Autodesk Inventor part; units mm, degrees
(part 2 of 2)
  spline S272 degree 2 poles (-165.9492, 93.5907) (-165.8958, 93.5647) (-165.7531, 93.5242) (-165.6883, 93.5242) knots 0 0 0 1 2 2 2
  spline S273 degree 2 poles (-165.6883, 93.5242) (-165.4922, 93.5242) (-165.2539, 93.8208) (-165.2539, 94.0915) knots 0 0 0 1 2 2 2
  spline S274 degree 2 poles (-165.2539, 94.0915) (-165.2539, 94.3557) (-165.4841, 94.6523) (-165.6883, 94.6523) knots 0 0 0 1 2 2 2
  spline S275 degree 2 poles (-165.6883, 94.6523) (-165.8115, 94.6523) (-166.0351, 94.5502) (-166.121, 94.4707) knots 0 0 0 1 2 2 2
  line L249 (-166.121, 94.4707) -> (-166.1356, 94.4707)
  line L250 (-166.1356, 94.4707) -> (-166.1356, 94.7544)
  spline S276 degree 2 poles (-166.1356, 94.7544) (-166.0984, 94.7722) (-165.9849, 94.8224) (-165.9395, 94.8338) knots 0 0 0 1 2 2 2
  spline S277 degree 2 poles (-165.9395, 94.8338) (-165.8747, 94.8532) (-165.7726, 94.8727) (-165.6932, 94.8727) knots 0 0 0 1 2 2 2
  spline S278 degree 2 poles (-167.2021, 94.6798) (-167.1713, 94.7025) (-167.0676, 94.7835) (-167.0189, 94.8079) knots 0 0 0 1 2 2 2
  spline S279 degree 2 poles (-167.0189, 94.8079) (-166.9525, 94.8435) (-166.8277, 94.8808) (-166.7142, 94.8808) knots 0 0 0 1 2 2 2
  spline S280 degree 2 poles (-166.7142, 94.8808) (-166.6219, 94.8808) (-166.4549, 94.8111) (-166.3917, 94.7479) knots 0 0 0 1 2 2 2
  spline S281 degree 2 poles (-166.3917, 94.7479) (-166.3317, 94.6863) (-166.2588, 94.5048) (-166.2588, 94.4043) knots 0 0 0 1 2 2 2
  spline S282 degree 2 poles (-166.2588, 94.4043) (-166.2588, 94.2487) (-166.3901, 94.0283) (-166.5327, 93.9651) knots 0 0 0 1 2 2 2
  spline S283 degree 2 poles (-166.5327, 93.9651) (-166.6591, 93.9067) (-167.0027, 93.863) (-167.2021, 93.8516) knots 0 0 0 1 2 2 2
  line L251 (-167.2021, 93.8516) -> (-167.2021, 93.803)
  spline S284 degree 2 poles (-167.2021, 93.803) (-167.2021, 93.7155) (-167.1486, 93.6069) (-167.1, 93.5761) knots 0 0 0 1 2 2 2
  spline S285 degree 2 poles (-167.1, 93.5761) (-167.0514, 93.5453) (-166.912, 93.5259) (-166.8374, 93.5259) knots 0 0 0 1 2 2 2
  spline S286 degree 2 poles (-166.8374, 93.5259) (-166.7499, 93.5259) (-166.5133, 93.5777) (-166.395, 93.628) knots 0 0 0 1 2 2 2
  line L252 (-166.395, 93.628) -> (-166.3804, 93.628)
  line L253 (-166.3804, 93.628) -> (-166.3804, 93.3703)
  spline S287 degree 2 poles (-166.3804, 93.3703) (-166.4501, 93.3508) (-166.711, 93.3022) (-166.839, 93.3022) knots 0 0 0 1 2 2 2
  spline S288 degree 2 poles (-166.839, 93.3022) (-166.9946, 93.3022) (-167.2069, 93.3508) (-167.2912, 93.414) knots 0 0 0 1 2 2 2
  spline S289 degree 2 poles (-167.2912, 93.414) (-167.3739, 93.4756) (-167.4549, 93.6717) (-167.4549, 93.8127) knots 0 0 0 1 2 2 2
  line L254 (-167.4549, 93.8127) -> (-167.4549, 94.8387)
  line L255 (-167.4549, 94.8387) -> (-167.2021, 94.8387)
  line L256 (-167.2021, 94.8387) -> (-167.2021, 94.6798)
  line L257 (-167.2021, 94.4691) -> (-167.2021, 94.0526)
  spline S290 degree 2 poles (-167.2021, 94.0526) (-167.1113, 94.0607) (-166.8374, 94.0882) (-166.7515, 94.1142) knots 0 0 0 1 2 2 2
  spline S291 degree 2 poles (-166.7515, 94.1142) (-166.651, 94.145) (-166.5197, 94.273) (-166.5197, 94.3865) knots 0 0 0 1 2 2 2
  spline S292 degree 2 poles (-166.5197, 94.3865) (-166.5197, 94.5161) (-166.6656, 94.6474) (-166.805, 94.6474) knots 0 0 0 1 2 2 2
  spline S293 degree 2 poles (-166.805, 94.6474) (-166.9233, 94.6474) (-167.1178, 94.5453) (-167.2021, 94.4691) knots 0 0 0 1 2 2 2
  line L258 (-169.5116, 94.8387) -> (-169.5116, 93.9699)
  spline S294 degree 2 poles (-169.5116, 93.9699) (-169.5116, 93.8662) (-169.4954, 93.6895) (-169.4695, 93.6409) knots 0 0 0 1 2 2 2
  spline S295 degree 2 poles (-169.4695, 93.6409) (-169.4436, 93.5874) (-169.3447, 93.5356) (-169.2588, 93.5356) knots 0 0 0 1 2 2 2
  spline S296 degree 2 poles (-169.2588, 93.5356) (-169.181, 93.5356) (-169.0027, 93.6312) (-168.9087, 93.722) knots 0 0 0 1 2 2 2
  spline S297 degree 2 poles (-168.9087, 93.722) (-168.9103, 93.7447) (-168.9136, 93.8079) (-168.9136, 93.85) knots 0 0 0 1 2 2 2
  line L259 (-168.9136, 93.85) -> (-168.9136, 94.8387)
  line L260 (-168.9136, 94.8387) -> (-168.6608, 94.8387)
  line L261 (-168.6608, 94.8387) -> (-168.6608, 93.9699)
  spline S298 degree 2 poles (-168.6608, 93.9699) (-168.6608, 93.8662) (-168.6445, 93.6895) (-168.6186, 93.6409) knots 0 0 0 1 2 2 2
  spline S299 degree 2 poles (-168.6186, 93.6409) (-168.5927, 93.5874) (-168.4938, 93.5356) (-168.4079, 93.5356) knots 0 0 0 1 2 2 2
  spline S300 degree 2 poles (-168.4079, 93.5356) (-168.3269, 93.5356) (-168.147, 93.6377) (-168.0627, 93.7171) knots 0 0 0 1 2 2 2
  line L262 (-168.0627, 93.7171) -> (-168.0627, 94.8387)
  line L263 (-168.0627, 94.8387) -> (-167.8099, 94.8387)
  line L264 (-167.8099, 94.8387) -> (-167.8099, 93.3378)
  line L265 (-167.8099, 93.3378) -> (-168.0627, 93.3378)
  line L266 (-168.0627, 93.3378) -> (-168.0627, 93.5032)
  spline S301 degree 2 poles (-168.0627, 93.5032) (-168.1616, 93.4043) (-168.3561, 93.2957) (-168.4727, 93.2957) knots 0 0 0 1 2 2 2
  spline S302 degree 2 poles (-168.4727, 93.2957) (-168.6056, 93.2957) (-168.8115, 93.4173) (-168.865, 93.555) knots 0 0 0 1 2 2 2
  spline S303 degree 2 poles (-168.865, 93.555) (-168.98, 93.427) (-169.1972, 93.2957) (-169.3236, 93.2957) knots 0 0 0 1 2 2 2
  spline S304 degree 2 poles (-169.3236, 93.2957) (-169.4209, 93.2957) (-169.5797, 93.3557) (-169.6381, 93.4237) knots 0 0 0 1 2 2 2
  spline S305 degree 2 poles (-169.6381, 93.4237) (-169.698, 93.4918) (-169.7645, 93.696) (-169.7645, 93.85) knots 0 0 0 1 2 2 2
  line L267 (-169.7645, 93.85) -> (-169.7645, 94.8387)
  line L268 (-169.7645, 94.8387) -> (-169.5116, 94.8387)
  spline S306 degree 2 poles (-170.771, 94.8727) (-170.4112, 94.8727) (-170.0157, 94.4691) (-170.0157, 94.0964) knots 0 0 0 1 2 2 2
  spline S307 degree 2 poles (-170.0157, 94.0964) (-170.0157, 93.7301) (-170.3998, 93.2957) (-170.7094, 93.2957) knots 0 0 0 1 2 2 2
  spline S308 degree 2 poles (-170.7094, 93.2957) (-170.8488, 93.2957) (-171.0643, 93.3767) (-171.1437, 93.4626) knots 0 0 0 1 2 2 2
  spline S309 degree 2 poles (-171.1437, 93.4626) (-171.2248, 93.5485) (-171.3107, 93.7965) (-171.3107, 93.9764) knots 0 0 0 1 2 2 2
  line L269 (-171.3107, 93.9764) -> (-171.3107, 94.1142)
  line L270 (-171.3107, 94.1142) -> (-170.2718, 94.1142)
  spline S310 degree 2 poles (-170.2718, 94.1142) (-170.2718, 94.3751) (-170.5343, 94.6523) (-170.7677, 94.6523) knots 0 0 0 1 2 2 2
  spline S311 degree 2 poles (-170.7677, 94.6523) (-170.8504, 94.6523) (-171.0108, 94.615) (-171.0757, 94.5858) knots 0 0 0 1 2 2 2
  spline S312 degree 2 poles (-171.0757, 94.5858) (-171.1437, 94.5534) (-171.2377, 94.4967) (-171.2685, 94.4707) knots 0 0 0 1 2 2 2
  line L271 (-171.2685, 94.4707) -> (-171.2831, 94.4707)
  line L272 (-171.2831, 94.4707) -> (-171.2831, 94.7463)
  spline S313 degree 2 poles (-171.2831, 94.7463) (-171.2394, 94.7641) (-171.1065, 94.816) (-171.0546, 94.8306) knots 0 0 0 1 2 2 2
  spline S314 degree 2 poles (-171.0546, 94.8306) (-170.9817, 94.8516) (-170.8617, 94.8727) (-170.771, 94.8727) knots 0 0 0 1 2 2 2
  spline S315 degree 2 poles (-171.0643, 93.9213) (-171.0611, 93.8192) (-171.0189, 93.6701) (-170.9784, 93.6199) knots 0 0 0 1 2 2 2
  spline S316 degree 2 poles (-170.9784, 93.6199) (-170.9347, 93.5631) (-170.7969, 93.5032) (-170.6948, 93.5032) knots 0 0 0 1 2 2 2
  spline S317 degree 2 poles (-170.6948, 93.5032) (-170.5943, 93.5032) (-170.4533, 93.5631) (-170.395, 93.6215) knots 0 0 0 1 2 2 2
  spline S318 degree 2 poles (-170.395, 93.6215) (-170.3382, 93.6814) (-170.2799, 93.8257) (-170.2718, 93.9213) knots 0 0 0 1 2 2 2
  line L273 (-170.2718, 93.9213) -> (-171.0643, 93.9213)
  line L274 (-172.3625, 93.6085) -> (-172.3496, 93.6085)
  spline S319 degree 2 poles (-172.3496, 93.6085) (-172.3204, 93.6004) (-172.2572, 93.5972) (-172.2134, 93.5972) knots 0 0 0 1 2 2 2
  spline S320 degree 2 poles (-172.2134, 93.5972) (-172.1113, 93.5972) (-171.9103, 93.6863) (-171.8196, 93.7738) knots 0 0 0 1 2 2 2
  line L275 (-171.8196, 93.7738) -> (-171.8196, 94.8387)
  line L276 (-171.8196, 94.8387) -> (-171.5668, 94.8387)
  line L277 (-171.5668, 94.8387) -> (-171.5668, 93.3378)
  line L278 (-171.5668, 93.3378) -> (-171.8196, 93.3378)
  line L279 (-171.8196, 93.3378) -> (-171.8196, 93.5615)
  spline S321 degree 2 poles (-171.8196, 93.5615) (-171.9573, 93.4383) (-172.1632, 93.3378) (-172.2604, 93.3378) knots 0 0 0 1 2 2 2
  spline S322 degree 2 poles (-172.2604, 93.3378) (-172.2993, 93.3378) (-172.3382, 93.3411) (-172.3625, 93.3459) knots 0 0 0 1 2 2 2
  line L280 (-172.3625, 93.3459) -> (-172.3625, 93.6085)
  spline S323 degree 2 poles (-173.395, 94.6798) (-173.3642, 94.7025) (-173.2604, 94.7835) (-173.2118, 94.8079) knots 0 0 0 1 2 2 2
  spline S324 degree 2 poles (-173.2118, 94.8079) (-173.1454, 94.8435) (-173.0206, 94.8808) (-172.9071, 94.8808) knots 0 0 0 1 2 2 2
  spline S325 degree 2 poles (-172.9071, 94.8808) (-172.8147, 94.8808) (-172.6478, 94.8111) (-172.5846, 94.7479) knots 0 0 0 1 2 2 2
  spline S326 degree 2 poles (-172.5846, 94.7479) (-172.5246, 94.6863) (-172.4517, 94.5048) (-172.4517, 94.4043) knots 0 0 0 1 2 2 2
  spline S327 degree 2 poles (-172.4517, 94.4043) (-172.4517, 94.2487) (-172.583, 94.0283) (-172.7256, 93.9651) knots 0 0 0 1 2 2 2
  spline S328 degree 2 poles (-172.7256, 93.9651) (-172.852, 93.9067) (-173.1956, 93.863) (-173.395, 93.8516) knots 0 0 0 1 2 2 2
  line L281 (-173.395, 93.8516) -> (-173.395, 93.803)
  spline S329 degree 2 poles (-173.395, 93.803) (-173.395, 93.7155) (-173.3415, 93.6069) (-173.2928, 93.5761) knots 0 0 0 1 2 2 2
  spline S330 degree 2 poles (-173.2928, 93.5761) (-173.2442, 93.5453) (-173.1048, 93.5259) (-173.0303, 93.5259) knots 0 0 0 1 2 2 2
  spline S331 degree 2 poles (-173.0303, 93.5259) (-172.9428, 93.5259) (-172.7061, 93.5777) (-172.5878, 93.628) knots 0 0 0 1 2 2 2
  line L282 (-172.5878, 93.628) -> (-172.5732, 93.628)
  line L283 (-172.5732, 93.628) -> (-172.5732, 93.3703)
  spline S332 degree 2 poles (-172.5732, 93.3703) (-172.6429, 93.3508) (-172.9039, 93.3022) (-173.0319, 93.3022) knots 0 0 0 1 2 2 2
  spline S333 degree 2 poles (-173.0319, 93.3022) (-173.1875, 93.3022) (-173.3998, 93.3508) (-173.4841, 93.414) knots 0 0 0 1 2 2 2
  spline S334 degree 2 poles (-173.4841, 93.414) (-173.5668, 93.4756) (-173.6478, 93.6717) (-173.6478, 93.8127) knots 0 0 0 1 2 2 2
  line L284 (-173.6478, 93.8127) -> (-173.6478, 94.8387)
  line L285 (-173.6478, 94.8387) -> (-173.395, 94.8387)
  line L286 (-173.395, 94.8387) -> (-173.395, 94.6798)
  line L287 (-173.395, 94.4691) -> (-173.395, 94.0526)
  spline S335 degree 2 poles (-173.395, 94.0526) (-173.3042, 94.0607) (-173.0303, 94.0882) (-172.9444, 94.1142) knots 0 0 0 1 2 2 2
  spline S336 degree 2 poles (-172.9444, 94.1142) (-172.8439, 94.145) (-172.7126, 94.273) (-172.7126, 94.3865) knots 0 0 0 1 2 2 2
  spline S337 degree 2 poles (-172.7126, 94.3865) (-172.7126, 94.5161) (-172.8585, 94.6474) (-172.9979, 94.6474) knots 0 0 0 1 2 2 2
  spline S338 degree 2 poles (-172.9979, 94.6474) (-173.1162, 94.6474) (-173.3107, 94.5453) (-173.395, 94.4691) knots 0 0 0 1 2 2 2
  point P0 (-22.6, -15.55)
  point P1 (-22.6, 4.75)
  point P2 (-22.6, 6.55)
  point P3 (-22.6, -17.35)
  point P4 (-20.8, -2.9403)
  point P5 (-20.8, -7.8597)
  point P6 (-3, 30.35)
  point P7 (-3, 59.1)
  point P8 (-105.5, 64)
  point P9 (-105.5, 64)
  point P10 (-120.5, 25.2)
  point P11 (-105.5, 25.2)
  point P12 (-147, -17)
  dimension "d0" = 190
  dimension "d1" = 100
  dimension "d2" = 3
  dimension "d14" = 5.4
  dimension "d15" = 10.25
  dimension "d16" = 42
  dimension "d17" = 4
  dimension "d18" = 10.5
  dimension "d19" = 42
  dimension "d20" = 4
  dimension "d21" = 4
  dimension "d31" = 110
  dimension "d32" = 30
  dimension "d33" = 53.8
  dimension "d34" = 7.5
  dimension "d35" = 7.5
  dimension "d64" = 6
  dimension "d65" = 6
  dimension "d66" = 6
  dimension "d67" = 6
  dimension "d68" = 6
  dimension "d69" = 6
  dimension "d70" = 6
  dimension "d71" = 6
  dimension "d85" = 22.5
  dimension "d86" = 10
  dimension "d87" = 20
  dimension "d88" = 6.5
  constraints: 124 end point, 25 equal length, 14 perpendicular, 13 horizontal, 12 point on line, 6 coincident, 5 midpoint, 4 symmetric about line, 2 other
  measures "d0" distance of L1.end L2.end
  measures "d1" distance of L0.end L1.end
  measures "d2" distance of L2.end L4.end
  measures "d14" distance of L6.start L6.end
  measures "d15" distance of L6.end L8.end
  measures "d16" distance of L11.end L10.end
  measures "d17" distance of L10.end L9.end
  measures "d18" distance of L6.end L13.end
  measures "d19" distance of L15.end L16.end
  measures "d20" distance of L14.end L15.end
  measures "d21" distance of L20.end L19.end
  measures "d31" distance of L6.end L22.end
  measures "d32" distance of L25.end L24.end
  measures "d33" distance of L24.end L23.end
  measures "d34" distance of L30.end L31.end
  measures "d35" distance of L29.end L30.end
  measures "d64" distance of L35.end L36.end
  measures "d65" distance of L34.end L35.end
  measures "d66" distance of L40.end L39.end
  measures "d67" distance of L39.end L38.end
  measures "d68" distance of L43.end L44.end
  measures "d69" distance of L42.end L43.end
  measures "d70" distance of L48.end L47.end
  measures "d71" distance of L47.end L46.end
  measures "d85" distance of L6.start L54.end
  measures "d86" distance of L54.end L55.end
  measures "d87" distance of L58.end L59.end
  measures "d88" distance of L57.end L58.end
extrude "Extrusion1" add sketch "Sketch1" along normal blind 10 contours L20 L12 L9 L19 L14 L17 L18 L3 | L11 L19 L9 L12 | L17 L14 L19 L16 | L11 L10 L9 L19 | L19 L14 L15 L16
sketch "Sketch2" plane through (-45, 30.35, 0) normal (0, -1, 0) x (1, 0, 0)
  line L0 (0, 10) -> (41, 10) construction
  line L1 (0, 10) -> (12.5, 10) construction
  line L2 (12.5, 10) -> (12.5, 5) construction
  line L3 (12.5, 5) -> (0, 5) construction
  line L4 (0, 5) -> (0, 10) construction
  circle A0 centre (12.5, 5) radius 1.35
  point P0 (45, 0)
  dimension "d24" = 12.5
  dimension "d25" = 5
  dimension "d26" = 2.7
  constraints: 8 end point, 2 parallel, 1 centre point, 1 coincident, 1 horizontal, 1 perpendicular
  measures "d24" distance of L2.end L3.end
  measures "d25" distance of L1.end L2.end
  measures "d26" diameter of A0
extrude "Extrusion2" cut sketch "Sketch2" against normal blind 30
extrude "Extrusion3" add sketch "Sketch1" against normal blind 2 contours L0 L1 L2 L3 L18 L16 L15 L51 L10 L11 L20 | L20 L12 L9 L19 L14 L17 L18 L3 | L11 L19 L9 L12 | L17 L14 L19 L16 | L11 L10 L9 L19 | L19 L14 L15 L16 | L9 L51 L14 L19 | L58 L59 L60 L61 | S0 S1 S2 S3 S4 S5 S6 S7 | S13 S12 S11 S10 S9 S8 | S14 S15 L66 L67 L68 L69 L70 S16 S17 | S21 S20 L71 S19 S18 | S22 S23 S24 S25 L72 L73 S26 S27 S28 L74 L75 S29 S30 | L76 S34 S33 S32 S31 | L77 L78 S35 S36 S37 L79 L80 L81 L82 L83 S38 S39 L84 | L85 L86 L87 L88 L89 L90 L91 L92 L93 L94 L95 L96 | L97 L98 L99 L100 L101 L102 L103 L104 | S40 S41 L105 L106 L107 L108 L109 S42 S43 | S47 S46 L110 S45 S44 | S48 S49 S50 S51 L111 L112 S52 S53 S54 L113 L114 S55 S56 | L115 S60 S59 S58 S57 | S61 S62 S63 S64 S65 S66 S67 S68 | S74 S73 S72 S71 S70 S69 | S75 S76 L116 L117 L118 L119 L120 S77 S78 | S82 S81 L121 S80 S79 | S83 S84 S85 S86 L122 L123 S87 S88 S89 L124 L125 S90 S91 | L126 S95 S94 S93 S92 | L127 L128 S96 S97 S98 L129 L130 L131 L132 L133 S99 S100 L134 | S101 L135 L136 S102 S103 S104 S105 S106 S107 S108 S109 S110 L137 L138 S111 S112 S113 S114 S115 S116 S117 | S118 S119 S120 S121 | S125 S124 S123 S122 | L139 L140 S126 S127 S128 L141 L142 L143 S129 S130 S131 L144 L145 L146 | L147 S132 S133 L148 L149 L150 L151 L152 S134 S135 L153 | S136 S137 S138 S139 S140 L154 L155 S141 S142 S143 S144 S145 L156 L157 S146 S147 | S148 S149 S150 S151 L158 L159 S152 S153 S154 L160 L161 S155 S156 | L162 S160 S159 S158 S157 | L163 L164 S161 S162 S163 L165 L166 L167 L168 L169 S164 S165 L170 | L171 L172 L173 L174 L175 L176 L177 L178 | S166 S167 L179 L180 L181 L182 L183 S168 S169 | S173 S172 L184 S171 S170 | S174 S175 S176 S177 L185 L186 S178 S179 S180 L187 L188 S181 S182 | L189 S186 S185 S184 S183 | L190 S187 S188 L191 L192 L193 L194 L195 S189 S190 L196 | S191 L197 L198 S192 S193 S194 S195 S196 S197 S198 S199 S200 L199 L200 S201 S202 S203 S204 S205 S206 S207 | S208 S209 L201 L202 L203 L204 L205 S210 S211 | S215 S214 L206 S213 S212 | S216 S217 S218 S219 L207 L208 S220 S221 S222 L209 L210 S223 S224 | L211 S228 S227 S226 S225 | S229 S230 S231 S232 S233 L212 L213 S234 S235 S236 S237 S238 L214 L215 S239 S240 | S241 L216 L217 L218 L219 L220 L221 L222 L223 L224 L225 L226 S242 S243 S244 L227 L228 S245 | L229 S246 S247 L230 L231 L232 L233 L234 S248 S249 L235 | S250 S251 S252 S253 S254 S255 L236 S256 S257 S258 L237 L238 S259 S260 S261 L239 L240 L241 | S265 S264 S263 S262 L242 | L243 L244 L245 L246 | S266 S267 S268 S269 S270 L247 L248 S271 S272 S273 S274 S275 L249 L250 S276 S277 | S278 S279 S280 S281 S282 S283 L251 S284 S285 S286 L252 L253 S287 S288 S289 L254 L255 L256 | S293 S292 S291 S290 L257 | L258 S294 S295 S296 S297 L259 L260 L261 S298 S299 S300 L262 L263 L264 L265 L266 S301 S302 S303 S304 S305 L267 L268 | S306 S307 S308 S309 L269 L270 S310 S311 S312 L271 L272 S313 S314 | L273 S318 S317 S316 S315 | L274 S319 S320 L275 L276 L277 L278 L279 S321 S322 L280 | S323 S324 S325 S326 S327 S328 L281 S329 S330 S331 L282 L283 S332 S333 S334 L284 L285 L286 | S338 S337 S336 S335 L287
hole "Hole1" at (-120.5, 64, 0) at (-105.5, 64, 0) at (-120.5, 25.2, 0) at (-105.5, 25.2, 0) direction (0, 0, -1) diameter 3 depth 5 tip angle 118
sketch "Sketch3" plane through (0, 0, -2) normal (0, 0, -1) x (-1, 0, 0)
  line L0 (0, 100) -> (0, 0) construction
  line L1 (0, 0) -> (20, 0) construction
  line L2 (20, 0) -> (20, 3.5) construction
  line L3 (20, 3.5) -> (0, 3.5) construction
  line L4 (0, 3.5) -> (0, 0) construction
  line L5 (20, 3.5) -> (170, 3.5)
  line L6 (170, 3.5) -> (170, 6.5)
  line L7 (170, 6.5) -> (20, 6.5)
  line L8 (20, 6.5) -> (20, 3.5)
  line L9 (0, 0) -> (0, 50) construction
  line L10 (0, 50) -> (190.5533, 50) construction
  line L11 (190, 0) -> (190, 100) construction
  line L12 (190, 0) -> (186.5, 0) construction
  line L13 (186.5, 0) -> (186.5, 20) construction
  line L14 (186.5, 20) -> (190, 20) construction
  line L15 (190, 20) -> (190, 0) construction
  line L16 (186.5, 20) -> (183.5, 20)
  line L17 (183.5, 20) -> (183.5, 80)
  line L18 (183.5, 80) -> (186.5, 80)
  line L19 (186.5, 80) -> (186.5, 20)
  line L20 (95.2766, 50) -> (95.2766, 0) construction
  line L21 (0, 0) -> (190, 0) construction
  line L22 (95.2766, 50) -> (145.2766, 50) construction
  line L23 (0, 100) -> (20, 100) construction
  line L24 (20, 100) -> (20, 96.5) construction
  line L25 (20, 96.5) -> (0, 96.5) construction
  line L26 (0, 96.5) -> (0, 100) construction
  line L27 (0, 100) -> (3.5, 100) construction
  line L28 (3.5, 100) -> (3.5, 80) construction
  line L29 (3.5, 80) -> (0, 80) construction
  line L30 (0, 80) -> (0, 100) construction
  line L31 (20, 96.5) -> (170, 96.5)
  line L32 (170, 96.5) -> (170, 93.5)
  line L33 (170, 93.5) -> (20, 93.5)
  line L34 (20, 93.5) -> (20, 96.5)
  line L35 (3.5, 80) -> (7, 80)
  line L36 (7, 80) -> (7, 20)
  line L37 (7, 20) -> (3.5, 20)
  line L38 (3.5, 20) -> (3.5, 80)
  dimension "d43" = 20
  dimension "d44" = 3.5
  dimension "d45" = 150
  dimension "d46" = 3
  dimension "d47" = 50
  dimension "d48" = 3.5
  dimension "d49" = 20
  dimension "d50" = 3
  dimension "d51" = 60
  dimension "d52" = 50
  dimension "d53" = 90
  dimension "d54" = 20
  dimension "d55" = 3.5
  dimension "d56" = 3.5
  dimension "d57" = 20
  dimension "d58" = 150
  dimension "d59" = 3
  dimension "d60" = 3.5
  dimension "d61" = 60
  constraints: 72 end point, 16 parallel, 11 perpendicular, 9 horizontal, 2 midpoint
  measures "d43" distance of L3.end L2.end
  measures "d44" distance of L2.end L1.end
  measures "d45" distance of L7.end L6.end
  measures "d46" distance of L6.end L5.end
  measures "d47" distance of L0.end L9.end
  measures "d48" distance of L13.end L14.end
  measures "d49" distance of L12.end L13.end
  measures "d50" distance of L17.end L18.end
  measures "d51" distance of L16.end L17.end
  measures "d52" distance of L20.start L20.end
  measures "d53" angle of L20 L22
  measures "d54" distance of L24.end L25.end
  measures "d55" distance of L23.end L24.end
  measures "d56" distance of L28.end L29.end
  measures "d57" distance of L27.end L28.end
  measures "d58" distance of L32.end L33.end
  measures "d59" distance of L31.end L32.end
  measures "d60" distance of L36.end L37.end
  measures "d61" distance of L35.end L36.end
extrude "Extrusion4" add sketch "Sketch3" along normal blind 2
hole "Hole2" at (-184, 94, 0) at (-6, 94, 0) at (-6, 6, 0) at (-184, 6, 0) direction (0, 0, -1) diameter 3 depth 6.5 tip angle 118 counterbore diameter 5.5 counterbore depth 1.5
fillet "Fillet1" radius 2 4 edges at (0, 0, -1) (-190, 0, -1) (-190, 100, -1) (0, 100, -1)
fillet "Fillet2" radius 2 9 edges at (-0.5858, 0.5858, 0) (0, 16.175, 0) (-189.4142, 0.5858, 0) (-190, 50, 0) (-189.4142, 99.4142, 0) (-95, 100, 0) (-0.5858, 99.4142, 0) (0, 78.55, 0) (-95, 0, 0)
fillet "Fillet3" radius 1 4 edges at (-95, 6.5, -2) (-183.5, 50, -2) (-95, 93.5, -2) (-7, 50, -2)
fillet "Fillet4" radius 1 2 edges at (-45, 57.1, 10) (-45, 32.35, 10)
extrude "Extrusion5" add sketch "Sketch1" along normal blind 1.8 contours L9 L51 L14 L19
extrude "Extrusion6" cut sketch "Sketch1" against normal blind 10 contours L58 L59 L60 L61
fillet "Fillet5" radius 2 4 edges at (-0.5858, 30.35, -0.5858) (-23.5, 30.35, 0) (-0.5858, 59.1, -0.5858) (-23.5, 59.1, 0)
extrude "Extrusion7" add sketch "Sketch1" along normal blind 0.5 contours S0 S1 S2 S3 S4 S5 S6 S7 | S14 S15 L66 L67 L68 L69 L70 S16 S17 | S22 S23 S24 S25 L72 L73 S26 S27 S28 L74 L75 S29 S30 | L77 L78 S35 S36 S37 L79 L80 L81 L82 L83 S38 S39 L84 | L85 L86 L87 L88 L89 L90 L91 L92 L93 L94 L95 L96 | L97 L98 L99 L100 L101 L102 L103 L104 | S40 S41 L105 L106 L107 L108 L109 S42 S43 | S48 S49 S50 S51 L111 L112 S52 S53 S54 L113 L114 S55 S56 | S61 S62 S63 S64 S65 S66 S67 S68 | S75 S76 L116 L117 L118 L119 L120 S77 S78 | S83 S84 S85 S86 L122 L123 S87 S88 S89 L124 L125 S90 S91 | L127 L128 S96 S97 S98 L129 L130 L131 L132 L133 S99 S100 L134 | S101 L135 L136 S102 S103 S104 S105 S106 S107 S108 S109 S110 L137 L138 S111 S112 S113 S114 S115 S116 S117 | S118 S119 S120 S121 | L139 L140 S126 S127 S128 L141 L142 L143 S129 S130 S131 L144 L145 L146 | L147 S132 S133 L148 L149 L150 L151 L152 S134 S135 L153 | S136 S137 S138 S139 S140 L154 L155 S141 S142 S143 S144 S145 L156 L157 S146 S147 | S148 S149 S150 S151 L158 L159 S152 S153 S154 L160 L161 S155 S156 | L163 L164 S161 S162 S163 L165 L166 L167 L168 L169 S164 S165 L170 | L171 L172 L173 L174 L175 L176 L177 L178 | S166 S167 L179 L180 L181 L182 L183 S168 S169 | S174 S175 S176 S177 L185 L186 S178 S179 S180 L187 L188 S181 S182 | L190 S187 S188 L191 L192 L193 L194 L195 S189 S190 L196 | S191 L197 L198 S192 S193 S194 S195 S196 S197 S198 S199 S200 L199 L200 S201 S202 S203 S204 S205 S206 S207 | S208 S209 L201 L202 L203 L204 L205 S210 S211 | S216 S217 S218 S219 L207 L208 S220 S221 S222 L209 L210 S223 S224 | S229 S230 S231 S232 S233 L212 L213 S234 S235 S236 S237 S238 L214 L215 S239 S240 | S241 L216 L217 L218 L219 L220 L221 L222 L223 L224 L225 L226 S242 S243 S244 L227 L228 S245 | L229 S246 S247 L230 L231 L232 L233 L234 S248 S249 L235 | S250 S251 S252 S253 S254 S255 L236 S256 S257 S258 L237 L238 S259 S260 S261 L239 L240 L241 | L243 L244 L245 L246 | S266 S267 S268 S269 S270 L247 L248 S271 S272 S273 S274 S275 L249 L250 S276 S277 | S278 S279 S280 S281 S282 S283 L251 S284 S285 S286 L252 L253 S287 S288 S289 L254 L255 L256 | L258 S294 S295 S296 S297 L259 L260 L261 S298 S299 S300 L262 L263 L264 L265 L266 S301 S302 S303 S304 S305 L267 L268 | S306 S307 S308 S309 L269 L270 S310 S311 S312 L271 L272 S313 S314 | L274 S319 S320 L275 L276 L277 L278 L279 S321 S322 L280 | S323 S324 S325 S326 S327 S328 L281 S329 S330 S331 L282 L283 S332 S333 S334 L284 L285 L286
fillet "Fillet6" radius 0.5 8 edges at (-35, 76, 0) (-45, 79.25, 0) (-35, 82.5, 0) (-25, 79.25, 0) (-35, 76, -2) (-35, 82.5, -2) (-25, 79.25, -2) (-45, 79.25, -2)
equation "\"d64\" = d65"
body "Solid1"
